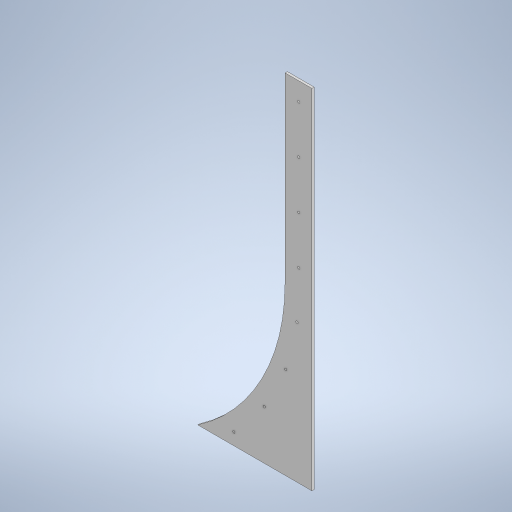
# Autodesk Inventor part: boundaryHalf1V1
Saved by Autodesk Inventor 2024.4 (Build 284460000, 460)
## iProperties
Created: 2025-11-05
Part Number: boundaryHalf1V1
Material: Generic
Document SubType Name: Modeling
Designer: jonas
Density: 1 g/cm^3
Appearance: Default
Author: jonas
Autodesk Inventor part; units mm, degrees
ref_plane "YZ Plane" through (0, 0, 0) normal (1, 0, 0) x (0, 1, 0)
ref_plane "XZ Plane" through (0, 0, 0) normal (0, 1, 0) x (-1, 0, 0)
ref_plane "XY Plane" through (0, 0, 0) normal (0, 0, 1) x (1, 0, 0)
sketch "Sketch1" plane through (0, 0, 0) normal (0, 1, 0) x (-1, 0, 0)
  line L0 (0, 290.198) -> (0, -290.198) construction
  line L1 (98.4779, 0) -> (-98.4779, 0) construction
  arc A0 (-441.1, 0) -> (-250, -363.4133) centre (0, 0) ccw
  line L2 (-441.1, 0) -> (-441.1, 400)
  line L3 (-441.1, 400) -> (-500, 400)
  line L4 (-500, 400) -> (-500, -363.4133)
  line L5 (-250, -363.4133) -> (-500, -363.4133)
  dimension "d0" = 500
  dimension "d1" = 400
  dimension "d3" = 441.1
  dimension "d5" = 363.4133
  constraints: 12 end point, 3 coincident, 2 horizontal, 2 midpoint, 2 perpendicular, 2 point on circle, 2 vertical, 1 centre point, 1 tangent
  measures "d0" distance between parallel lines of L4 L0
  measures "d1" distance between parallel lines of L3 L1
  measures "d3" radius of A0
  measures "d5" distance between parallel lines of L1 L5
extrude "Extrusion1" add sketch "Sketch1" along normal blind 5
sketch "Sketch2" plane through (0, 0, 0) normal (0, -1, 0) x (1, 0, 0)
  line L0 (441.1, 400) -> (500, 400) projected
  line L1 (441.1, 0) -> (441.1, 400) projected
  line L2 (0, 0) -> (467.2725, -59.9302) construction
  line L3 (0, 0) -> (442.392, -161.9398) construction
  line L4 (0, 0) -> (395.535, -255.9048) construction
  line L5 (0, 0) -> (329.0291, -337.1573) construction
  line L6 (471.1, 255) -> (471.1, 360) construction
  line L7 (471.1, 255) -> (471.1, 150) construction
  line L8 (471.1, 150) -> (471.1, 45) construction
  line L9 (500, 400) -> (500, -363.4133) construction
  line L10 (471.1, 45) -> (467.2725, -59.9302) construction
  line L11 (467.2725, -59.9302) -> (442.392, -161.9398) construction
  line L12 (442.392, -161.9398) -> (395.535, -255.9048) construction
  line L13 (395.535, -255.9048) -> (329.0291, -337.1573) construction
  point P0 (470.55, 400)
  dimension "d8" = 40
  dimension "d9" = 30
  dimension "d10" = 471.1
  dimension "d15" = 105
  constraints: 22 end point, 9 equal length, 3 vertical alignment, 2 vertical, 1 midpoint, 1 parallel
  measures "d8" vertical distance of point (470.55, 400) L6.end
  measures "d9" distance from line of L1 L6.end
  measures "d10" distance of L2.start L2.end
  measures "d15" distance of L6.start L6.end
hole "Hole1" at (471.1, 0, 360) at (471.1, 0, 255) at (471.1, 0, 150) at (471.1, 0, 45) at (467.2725, 0, -59.9302) at (442.392, 0, -161.9398) at (395.535, 0, -255.9048) at (329.0291, 0, -337.1573) direction (0, 1, 0) diameter 5 end through all
body "Solid1"
